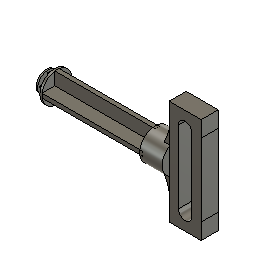
jeringuilla_scotchshort (Autodesk Fusion 360 design; units mm, degrees)
part number: 2026-03-25-12-15-58-128
Autodesk Fusion 360 part; units mm, degrees
sketch "Boceto1" plane through (0, 0, 0) normal (1, 0, 0) x (0, 0, -1)
  circle A0 centre (0, 0) radius 5
  dimension "d1" = 10
  constraint coincident A0.centre origin
  measures "d1" diameter of A0
extrude "Extruir1" add sketch "Boceto1" along normal blind 1 makes body 1
sketch "Boceto2" plane through (1, 0, 0) normal (1, 0, 0) x (0, 0, -1)
  circle A0 centre (0, 0) radius 5
  line L0 (-4, 0) -> (4, 0)
  line L1 (4, 0) -> (4, 0.5)
  line L2 (4, 0.5) -> (0.5, 0.5)
  line L3 (0.5, 0.5) -> (0.5, 4)
  line L4 (0.5, 4) -> (-0.5, 4)
  line L5 (-0.5, 4) -> (-0.5, 0.5)
  line L6 (-0.5, 0.5) -> (-4, 0.5)
  line L7 (-4, 0.5) -> (-4, 0)
  line L8 (0, 4) -> (0, 0)
  line L9 (0.5, -4) -> (-0.5, -4)
  line L10 (-0.5, -4) -> (-0.5, -0.5)
  line L11 (0.5, -0.5) -> (0.5, -4)
  line L12 (-0.5, -0.5) -> (-4, -0.5)
  line L13 (-4, -0.5) -> (-4, 0)
  line L14 (4, -0.5) -> (0.5, -0.5)
  line L15 (4, 0) -> (4, -0.5)
  dimension "d74" = 1
  dimension "d75" = 0.5
  dimension "d76" = 0.5
  dimension "d77" = 4
  dimension "d78" = 4
  dimension "d79" = 4
  constraint horizontal L0
  constraint perpendicular L0 L1
  constraint perpendicular L1 L2
  constraint perpendicular L2 L3
  constraint perpendicular L3 L4
  constraint perpendicular L4 L5
  constraint perpendicular L5 L6
  constraint perpendicular L0 L7
  constraint midpoint L4 L8.start
  constraint coincident L0 A0.centre
  constraint perpendicular L0 L8
  constraint coincident A0.centre L8.end
  constraint symmetric L7.end L0 L13.end
  constraint symmetric L1.start L0 L15.start
  constraint symmetric L0 L1.end L14.start
  constraint symmetric L0 L2.end L11.start
  constraint symmetric L0 L3.end L9.start
  constraint symmetric L0 L4.end L9.end
  constraint symmetric L0 L5.end L10.end
  constraint symmetric L0 L6.end L12.end
  measures "d74" distance of L3.end L4.end
  measures "d75" distance of L0.end L1.end
  measures "d76" distance of L0.start L6.end
  measures "d77" distance of A0.centre L4
  measures "d78" distance of A0.centre L0.end
  measures "d79" distance of A0.centre L0.start
extrude "Extruir2" add sketch "Boceto2" along normal blind 3 contours L0 L4 L5 L6 L7 L8 | L0 L9 L10 L11 L12 L13 L14 L15 | L0 L1 L2 L3 L4 L8 bodies 1
sketch "Boceto3" plane through (4, 0, 0) normal (1, 0, 0) x (0, 0, -1)
  circle A0 centre (0, 0) radius 7
  line L0 (-4, 0.5) -> (-4, -0.5)
  line L1 (-4, -0.5) -> (-0.5, -0.5)
  line L2 (-0.5, -0.5) -> (-0.5, -4)
  line L3 (-0.5, -4) -> (0.5, -4)
  line L4 (0.5, -4) -> (0.5, -0.5)
  line L5 (0.5, -0.5) -> (4, -0.5)
  line L6 (4, -0.5) -> (4, 0.5)
  line L7 (4, 0.5) -> (0.5, 0.5)
  line L8 (0.5, 0.5) -> (0.5, 4)
  line L9 (0.5, 4) -> (-0.5, 4)
  line L10 (-0.5, 4) -> (-0.5, 0.5)
  line L11 (-0.5, 0.5) -> (-4, 0.5)
  dimension "d10" = 14
  constraint coincident A0.centre origin
  measures "d10" diameter of A0
extrude "Extruir3" add sketch "Boceto3" along normal blind 1 separate body contours A0 | L0 L1 L2 L3 L4 L5 L6 L7 L8 L9 L10 L11 makes body 2
sketch "Boceto4" plane through (5, 0, 0) normal (1, 0, 0) x (0, 0, -1)
  circle A0 centre (0, 0) radius 7
  line L0 (0, 7) -> (-1, 7)
  line L1 (-1, 7) -> (-1, 1)
  line L2 (-1, 1) -> (-7, 1)
  line L3 (-7, 1) -> (-7, -1)
  line L4 (-7, -1) -> (-1, -1)
  line L5 (-1, -1) -> (-1, -7)
  line L6 (-1, -7) -> (0, -7)
  line L7 (7, 0.5) -> (7, -0.5)
  line L8 (0, 7) -> (1, 7)
  line L9 (1, 7) -> (1, 1)
  line L10 (1, 1) -> (7, 1)
  line L11 (7, 1) -> (7, -1)
  line L12 (7, -1) -> (1, -1)
  line L13 (1, -1) -> (1, -7)
  line L14 (0, -7) -> (1, -7)
  dimension "d14" = 14
  dimension "d15" = 7
  dimension "d17" = 1
  dimension "d80" = 1
  dimension "d81" = 1
  dimension "d82" = 7
  constraint perpendicular L0 L1
  constraint perpendicular L2 L3
  constraint perpendicular L4 L5
  constraint perpendicular L13 L14
  measures "d14" distance of L0 L6
  measures "d15" distance of A0.centre L0
  measures "d17" distance of A0.centre L2
  measures "d80" distance of A0.centre L4
  measures "d81" distance of A0.centre L5
  measures "d82" distance of A0.centre L3
extrude "Extruir4" add sketch "Boceto4" along normal blind 47 contours A0 L1 L2 L4 L5 L9 L10 L12 L13 | A0 L7 L11 L12 | A0 L7 L10 L11 | A0 L8 L9 | A0 L13 L14 | A0 L0 L1 | A0 L5 L6 | A0 L2 L3 | A0 L3 L4 bodies 2
sketch "Boceto5" plane through (0, 0, 0) normal (0, 0, 1) x (1, 0, 0)
  circle A0 centre (62.3562, 0) radius 12.5
  circle A1 centre (62.3562, 0) radius 6
  line L0 (108, 14) -> (108, -14)
  point P0 (52, -7)
  point P1 (52, 7)
  dimension "d22" = 25
  dimension "d23" = 12
  constraint coincident A0 P0
  constraint coincident A0 P1
  constraint concentric A0 A1
  constraint vertical L0
  measures "d22" diameter of A0
  measures "d23" diameter of A1
sketch "Boceto9" plane through (0, 0, 0) normal (0, 0, 1) x (1, 0, 0)
  line L0 (114.4086, 19.3235) -> (112.7354, 19.3235)
  line L1 (109.7354, -21.184) -> (109.7958, -21.184)
  line L2 (101.5918, 19.3231) -> (103.2646, 19.3231)
  line L3 (100.2646, -21.184) -> (100.2042, -21.184)
  line L4 (125, 0.0018) -> (91.9611, 0.0018)
  line L5 (115.5, 17) -> (115.5, 0.0018)
  line L6 (115.5, 0.0018) -> (100.5, 0.0018)
  arc A0 (111.15, 17.0001) -> (104.85, 17.0061) centre (108, 17) ccw
  line L7 (111.15, 17.0001) -> (111.15, 0.0018)
  line L8 (104.85, 17.0061) -> (104.85, 0.0018)
  spline S0 degree 5 poles (100.5, 17) (100.5187, 16.549) (100.5236, 15.663) (100.4335, 14.3821) (100.1349, 12.7628) (99.5496, 10.8494) (98.847, 9.0066) (98.0997, 7.2067) (97.33, 5.4475) (96.4722, 3.7692) (95.4039, 2.2399) (94.2683, 1.1966) (93.2041, 0.5448) (92.3924, 0.1724) (91.9611, 0.0018) knots 0 0 0 0 0 0 0.1 0.2 0.3 0.4 0.5 0.6 0.7 0.8 0.9 1 1 1 1 1 1
  line L9 (100.384, 19.7975) -> (100.616, 14.2025)
  arc A1 (104.85, -17.0025) -> (111.15, -16.9965) centre (108, -16.9964) ccw
  line L10 (115.5, -16.9964) -> (115.5, 0.0018)
  line L11 (111.15, -16.9965) -> (111.15, 0.0018)
  line L12 (104.85, -17.0025) -> (104.85, 0.0018)
  spline S1 degree 5 poles (100.5, -16.9964) (100.5187, -16.5454) (100.5236, -15.6594) (100.4335, -14.3785) (100.1349, -12.7593) (99.5496, -10.8458) (98.847, -9.003) (98.0997, -7.2031) (97.33, -5.4439) (96.4722, -3.7657) (95.4039, -2.2364) (94.2683, -1.193) (93.2041, -0.5412) (92.3924, -0.1688) (91.9611, 0.0018) knots 0 0 0 0 0 0 0.1 0.2 0.3 0.4 0.5 0.6 0.7 0.8 0.9 1 1 1 1 1 1
  line L13 (94.7037, 1.0866) -> (89.2185, -1.083)
  line L14 (100.384, -19.7939) -> (100.616, -14.1989)
  line L15 (94.7037, -1.083) -> (89.2185, 1.0866)
  line L16 (115.5, 17) -> (115.5, 24.5)
  line L17 (115.5, 24.5) -> (100.5, 24.5)
  line L18 (100.5, 24.5) -> (100.5, 17)
  line L19 (115.5, -16.9964) -> (115.5, -24.5)
  line L20 (115.5, -24.5) -> (100.5, -24.5)
  line L21 (100.5, -24.5) -> (100.5, -16.9964)
  point P0 (98, 7)
  point P1 (98, -6.9964)
  point P2 (52, -7)
  dimension "d45" = 6.3
  constraint horizontal L0
  constraint horizontal L2
  constraint horizontal L4
  constraint coincident L4 L6.end
  constraint coincident L4 L5.end
  constraint perpendicular L4 L5
  constraint coincident L4 L7.end
  constraint coincident L6 L8.end
  constraint midpoint S0.start L9
  constraint midpoint L4.end L13
  constraint symmetric S0.end L4 S1.end
  constraint symmetric L4 L5.start L10.start
  constraint symmetric L4 L5.end L6.start
  constraint symmetric L4 S0.start S1.start
  constraint symmetric L4 A0.start A1.end
  constraint symmetric L4 A0.end A1.start
  constraint symmetric L4 A0 A1
  constraint symmetric L4 L7.end L11.end
  constraint symmetric L4 L8.end L12.end
  constraint symmetric L4 P0 P1
  constraint symmetric L4 L9.start L14.start
  constraint symmetric L4 L9.end L14.end
  constraint symmetric L4 L13.start L15.start
  constraint symmetric L4 L13.end L15.end
  constraint vertical L7
  constraint vertical L8
  constraint parallel L16 L18
  constraint parallel L19 L21
  measures "d45" diameter of A0
extrude "Extruir9" add sketch "Boceto9" along normal blind 4 and the other way blind 4 separate body contours L4 L6 A1 L10 L11 L12 S1 L19 L20 L21 | L4 L5 L6 A0 L7 L8 S0 L16 L17 L18 makes body 3
sketch "Boceto11" plane through (0, 0, 0) normal (0, 1, 0) x (1, 0, 0)
  spline S0 degree 5 poles (97.9999, 3.4935) (97.2252, 3.4915) (95.8142, 3.5439) (94.1126, 3.7919) (92.5545, 4.4019) (91.3618, 5.3875) (90.7293, 6.1571) (90.3396, 6.6313) (90.1084, 6.8871) (90, 7) knots 0 0 0 0 0 0 0.2 0.4 0.6 0.8 1 1 1 1 1 1
  line L0 (101.9999, 3.5039) -> (93.9999, 3.4831)
  line L1 (79, 0) -> (98, 0)
  line L2 (90, 7) -> (100.5, 7)
  line L3 (100.5, 7) -> (100.5, 3.5)
  line L4 (97.9999, 3.4935) -> (100.5, 3.5)
  spline S1 degree 5 poles (97.9999, -3.4935) (97.2252, -3.4915) (95.8142, -3.5439) (94.1126, -3.7919) (92.5545, -4.4019) (91.3618, -5.3875) (90.7293, -6.1571) (90.3396, -6.6313) (90.1084, -6.8871) (90, -7) knots 0 0 0 0 0 0 0.2 0.4 0.6 0.8 1 1 1 1 1 1
  line L5 (90.5624, 6.4147) -> (89.4376, 7.5853)
  line L6 (101.9999, -3.5039) -> (93.9999, -3.4831)
  line L7 (90.5624, -6.4147) -> (89.4376, -7.5853)
  line L8 (90, -7) -> (100.5, -7)
  line L9 (100.5, -7) -> (100.5, -3.5)
  line L10 (97.9999, -3.4935) -> (100.5, -3.5)
  line L11 (90, -7) -> (90, -10)
  line L12 (90, -10) -> (100.5, -10)
  line L13 (100.5, -10) -> (100.5, -7)
  line L14 (100.5, -4) -> (93.8398, -4)
  constraint midpoint S0.start L0
  constraint horizontal L1
  constraint horizontal L2
  constraint perpendicular L2 L3
  constraint midpoint S0.end L5
  constraint symmetric S0.start L1 S1.start
  constraint symmetric S0.end L1 S1.end
  constraint symmetric L0.start L1 L6.start
  constraint symmetric L0.end L1 L6.end
  constraint symmetric L1 L2.end L8.end
  constraint symmetric L1 L3.end L9.end
  constraint symmetric L1 L5.start L7.start
  constraint symmetric L1 L5.end L7.end
  constraint perpendicular L8 L11
  constraint perpendicular L11 L12
  constraint perpendicular L8 L13
  constraint coincident L9 L14.start
  constraint coincident S1 L14.end
  constraint perpendicular L9 L14
extrude "Extruir10" cut sketch "Boceto11" along normal through all and the other way through all bodies 2 3
sketch "Boceto15" plane through (0, 0, 0) normal (1, 0, 0) x (0, 0, -1)
  circle A0 centre (0, 0) radius 7.25
  dimension "d84" = 14.5
  constraint coincident A0.centre origin
  measures "d84" diameter of A0
extrude "Extruir12" add sketch "Boceto15" along normal blind 10.5 from surface at 90 bodies 3 2
move_body "Desplazar1" bodies 3 to x (1, 0, 0) y (0, 1, 0) z (0, 0, 1) at (-39, 0, 0)
chamfer "Chaflán1" distance 1 distance2 0.3 1 edges at (0, -1.8081, 4.6616) measured on face at (0.6667, -0.2492, -4.9938) on bodies 1
